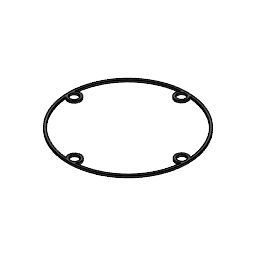
Gasket (Autodesk Fusion 360 design; units mm, degrees)
Autodesk Fusion 360 part; units mm, degrees
note: some values were not read from the file. Set by a fixed rule: which sketch regions a step uses.
sketch "Sketch1" plane through (0, 0, 0) normal (0, 1, 0) x (1, 0, 0)
  circle A0 centre (0, 0) radius 72.5
  circle A1 centre (0, 0) radius 70
  line L0 (-72.4995, -0.2589) -> (-64.9995, -0.2589)
  circle A2 centre (-64.9995, -0.2589) radius 7.5
  circle A3 centre (-64.9995, -0.2589) radius 5
  circle A4 centre (0.2589, -64.9995) radius 5
  circle A5 centre (0.2589, -64.9995) radius 7.5
  circle A6 centre (64.9995, 0.2589) radius 5
  circle A7 centre (64.9995, 0.2589) radius 7.5
  circle A8 centre (-0.2589, 64.9995) radius 5
  circle A9 centre (-0.2589, 64.9995) radius 7.5
  dimension "d1" = 145
  dimension "d2" = 140
  dimension "d3" = 7.5
  dimension "d4" = 15
  dimension "d5" = 10
  dimension "d7" = 360
  constraint coincident A0.centre A1.centre
  constraint concentric A0 A1
  constraint coincident A0 L0.start
  constraint horizontal L0
  constraint coincident L0.end A2.centre
  constraint concentric A2 A3
  measures "d1" diameter of A0
  measures "d2" diameter of A1
  measures "d3" distance of L0.start L0.end
  measures "d4" diameter of A2
  measures "d5" diameter of A3
extrude "Extrude1" add sketch "Sketch1" along normal blind 2 contours A0 A1 A6 A7 | A1 L0 A2 | A0 A1 A5 A7 | A0 A1 A7 A9 | A0 A1 A2 A9 | A1 L0 A2 | A0 A1 A2 A5 | A1 A5 | A1 A6 A7 | A1 A9 | A1 A5 | A1 A9 | A1 A2
